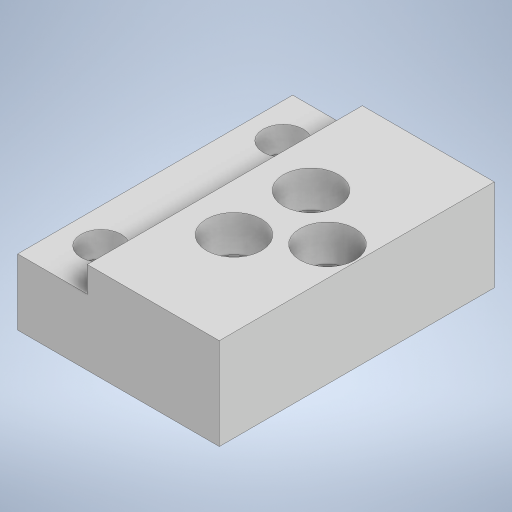
# Autodesk Inventor part: Feste Backe
Saved by Autodesk Inventor 2023 (Build 270158000, 158)
## iProperties
Created: 2023-05-10
Part Number: Feste Backe
Material: Generic
Document SubType Name: Modeling
Designer: dell
Density: 1 g/cm^3
Appearance: Default
Author: dell
Autodesk Inventor part; units mm, degrees
ref_plane "YZ Plane" through (0, 0, 0) normal (1, 0, 0) x (0, 1, 0)
ref_plane "XZ Plane" through (0, 0, 0) normal (0, 1, 0) x (-1, 0, 0)
ref_plane "XY Plane" through (0, 0, 0) normal (0, 0, 1) x (1, 0, 0)
sketch "Sketch1" plane through (0, 0, 0) normal (0, 1, 0) x (-1, 0, 0)
  line L0 (27.5, 37.5) -> (-27.5, 37.5)
  line L1 (-27.5, 37.5) -> (-27.5, -37.5)
  line L2 (-27.5, -37.5) -> (27.5, -37.5)
  line L3 (27.5, -37.5) -> (27.5, 37.5)
  line L4 (27.5, 37.5) -> (-27.5, -37.5) construction
  line L5 (-27.5, 37.5) -> (27.5, -37.5) construction
  point P0 (0, 0)
  dimension "d0" = 75
  dimension "d1" = 55
  constraints: 12 end point, 2 midpoint, 2 parallel, 1 horizontal, 1 perpendicular
  measures "d0" distance of L2.end L0.start
  measures "d1" distance of L1.end L2.end
extrude "Extrusion1" add sketch "Sketch1" along normal blind 18
sketch "Sketch2" plane through (0, 18, 0) normal (0, 1, 0) x (1, 0, 0)
  line L0 (-27.5, -37.5) -> (27.5, -37.5) projected
  line L1 (-8.5, -37.5) -> (-8.5, 37.5)
  line L2 (27.5, -37.5) -> (27.5, 37.5) projected
  line L3 (-8.5, 37.5) -> (27.5, 37.5)
  line L4 (-8.5, -37.5) -> (27.5, -37.5)
  dimension "d4" = 36
  constraints: 6 end point, 1 collinear, 1 horizontal, 1 point on line, 1 vertical
  measures "d4" distance of L1.end L2.end
extrude "Extrusion2" add sketch "Sketch2" along normal blind 7
sketch "Sketch3" plane through (0, 18, 0) normal (0, 1, 0) x (1, 0, 0)
  line L0 (27.5, 37.5) -> (-27.5, 37.5) projected
  line L1 (-27.5, 37.5) -> (-27.5, -37.5) projected
  line L2 (-8.5, 37.5) -> (-8.5, -37.5) projected
  circle A0 centre (-18, 25.4407) radius 5.5
  circle A1 centre (-18, -24.214) radius 5.5
  point P0 (0, 0)
  dimension "d9" = 19
  dimension "d10" = 11
  dimension "d11" = 11
  constraints: 2 centre point
  measures "d9" distance between parallel lines of L2 L1
  measures "d10" diameter of A0
  measures "d11" diameter of A1
extrude "Extrusion3" cut sketch "Sketch3" against normal blind 7
sketch "Sketch4" plane through (-18, 11, -25.4407) normal (0, 1, 0) x (1, 0, 0)
  circle A0 centre (0, 0) radius 3.2
  circle A1 centre (0, -49.6547) radius 5.5 projected
  circle A2 centre (0, -49.6547) radius 3.2
  point P0 (18, -25.4407)
  dimension "d14" = 6.4
  dimension "d15" = 6.4
  constraints: 2 centre point, 1 coincident
  measures "d14" diameter of A0
  measures "d15" diameter of A2
extrude "Extrusion4" cut sketch "Sketch4" against normal blind 15 contours A0 | A2
sketch "Sketch5" plane through (0, 25, 0) normal (0, 1, 0) x (1, 0, 0)
  circle A0 centre (19.5, 0) radius 7.5
  circle A1 centre (4.5, 10.5) radius 7.5
  circle A2 centre (4.5, -10.5) radius 7.5
  line L0 (27.5, -37.5) -> (27.5, 37.5) projected
  point P0 (0, 0)
  dimension "d18" = 15
  dimension "d19" = 15
  dimension "d20" = 15
  dimension "d21" = 23
  dimension "d22" = 23
  dimension "d23" = 8
  dimension "d26" = 21
  dimension "d27" = 10.5
  dimension "d28" = 10.5
  constraints: 3 centre point
  measures "d18" diameter of A1
  measures "d19" diameter of A0
  measures "d20" diameter of A2
  measures "d21" distance from line of L0 A1.centre
  measures "d22" distance from line of L0 A2.centre
  measures "d23" distance from line of L0 A0.centre
  measures "d26" distance of A2.centre A1.centre
  measures "d27" vertical distance of point (0, 0) A1.centre
  measures "d28" vertical distance of point (0, 0) A2.centre
extrude "Extrusion5" cut sketch "Sketch5" against normal blind 10
sketch "Sketch6" plane through (4.5, 15, 10.5) normal (0, 1, 0) x (1, 0, 0)
  circle A0 centre (0, 0) radius 4.2
  circle A1 centre (0, 21) radius 7.5 projected
  circle A2 centre (0, 21) radius 4.2
  circle A3 centre (15, 10.5) radius 7.5 projected
  circle A4 centre (15, 10.5) radius 4.2
  point P0 (-4.5, 10.5)
  dimension "d29" = 8.4
  dimension "d30" = 8.4
  dimension "d31" = 8.4
  constraints: 3 centre point, 2 coincident
  measures "d29" diameter of A0
  measures "d30" diameter of A2
  measures "d31" diameter of A4
extrude "Extrusion6" cut sketch "Sketch6" against normal blind 20 contours A0 | A2 | A4
body "Solid1"
